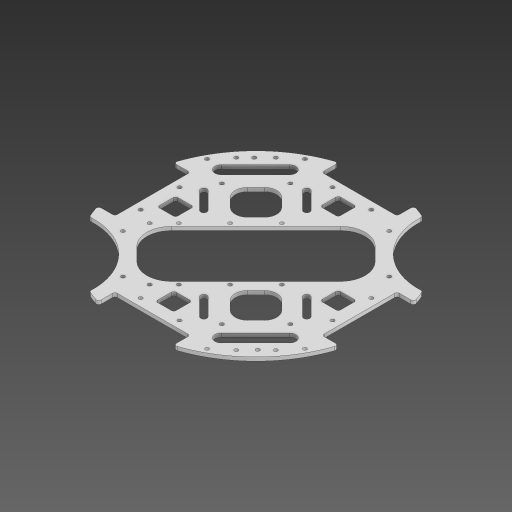
# Autodesk Inventor part: top
Saved by Autodesk Inventor 2023 (Build 270158000, 158)
## iProperties
Created: 2025-06-24
Part Number: top
Material: Типовые
Document SubType Name: Modeling
Designer: daa
Density: 1 g/cm^3
Appearance: По умолчанию
Author: daa
Autodesk Inventor part; units mm, degrees
ref_plane "YZ Plane" through (0, 0, 0) normal (1, 0, 0) x (0, 1, 0)
ref_plane "XZ Plane" through (0, 0, 0) normal (0, 1, 0) x (-1, 0, 0)
ref_plane "XY Plane" through (0, 0, 0) normal (0, 0, 1) x (1, 0, 0)
sketch "Эскиз1" plane through (0, 0, 0) normal (0, 1, 0) x (-1, 0, 0)
  line L0 (-79, -47.2724) -> (-79, 14.7276)
  line L1 (91.5447, -47.2724) -> (91.5447, 14.7276)
  line L2 (-79, -47.2724) -> (-93, -47.2724)
  line L3 (-79, 14.7276) -> (-93, 14.7276)
  line L4 (91.5447, -47.2724) -> (105.5447, -47.2724)
  line L5 (91.5447, 14.7276) -> (105.5447, 14.7276)
  line L6 (-24.7276, -101.5447) -> (37.2724, -101.5447)
  line L7 (-24.7276, 69) -> (37.2724, 69)
  line L8 (-24.7276, 69) -> (-24.7276, 83)
  line L9 (37.2724, 69) -> (37.2724, 83)
  line L10 (37.2724, -101.5447) -> (37.2724, -115.5447)
  line L11 (-24.7276, -101.5447) -> (-24.7276, -115.5447)
  arc A0 (-93, -47.2724) -> (-24.7276, -115.5447) centre (6.2724, -16.2724) ccw
  arc A1 (105.5447, 14.7276) -> (37.2724, 83) centre (6.2724, -16.2724) ccw
  arc A2 (-24.7276, 83) -> (-93, 14.7276) centre (6.2724, -16.2724) ccw
  arc A3 (37.2724, -115.5447) -> (105.5447, -47.2724) centre (6.2724, -16.2724) ccw
  dimension "d29" = 62
  dimension "d31" = 62
  dimension "d33" = 14
  dimension "d34" = 14
  dimension "d35" = 62
  dimension "d36" = 62
  dimension "d39" = 14
  dimension "d40" = 14
  constraints: 24 end point, 8 point on circle, 4 centre point, 4 horizontal, 3 parallel, 3 vertical, 2 point on line, 1 concentric
  measures "d29" distance of L0.start L0.end
  measures "d31" distance of L1.start L1.end
  measures "d33" distance of L0.end L3.end
  measures "d34" distance of L1.end L5.end
  measures "d35" distance of L6.start L6.end
  measures "d36" distance of L7.start L7.end
  measures "d39" distance of L7.start L8.end
  measures "d40" distance of L6.start L11.end
extrude "motor" add sketch "Эскиз1" along normal blind 3
sketch "Эскиз2" plane through (0, 3, 0) normal (0, 1, 0) x (1, 0, 0)
  arc A0 (24.7276, -83) -> (93, -14.7276) centre (-6.2724, 16.2724) ccw projected
  arc A1 (-37.2724, 115.5447) -> (-105.5447, 47.2724) centre (-6.2724, 16.2724) ccw projected
  circle A2 centre (-6.2724, 16.2724) radius 104
  line L0 (-6.2724, 16.2724) -> (-6.2724, -50.7276)
  arc A3 (-37.2724, 115.5447) -> (-105.5447, 47.2724) centre (-6.2724, 16.2724) ccw projected
  line L1 (-88.7917, -14.3063) -> (-40.8426, -62.2554)
  line L2 (-101.3809, -25.8032) -> (-48.3479, -78.8362)
  arc A4 (-105.5447, -14.7276) -> (-37.2724, -83) centre (-6.2724, 16.2724) ccw projected
  arc A5 (-48.3479, -78.8362) -> (-101.3809, -25.8032) centre (-98.035, -75.4903) ccw
  arc A6 (24.7276, -83) -> (93, -14.7276) centre (-6.2724, 16.2724) ccw projected
  line L3 (-79.8115, 89.8115) -> (67.2668, -57.2668)
  line L4 (24.3063, 98.7917) -> (72.2554, 50.8426)
  line L5 (35.8032, 111.3809) -> (88.8362, 58.3479)
  arc A7 (93, 47.2724) -> (24.7276, 115.5447) centre (-6.2724, 16.2724) ccw
  arc A8 (35.8032, 111.3809) -> (88.8362, 58.3479) centre (85.4903, 108.035) ccw
  line L6 (-91.5447, -14.7276) -> (-105.5447, -14.7276) projected
  arc A9 (-105.5447, -14.7276) -> (-101.3809, -25.8032) centre (-6.2724, 16.2724) ccw
  line L7 (-105.5447, -14.7276) -> (-80, -14.7276)
  point P0 (0, 0)
  point P1 (-6.2724, -50.7276)
  dimension "d181" = 208
  dimension "d190" = 67
  dimension "d205" = 75
  dimension "d207" = 17.0315
  dimension "d208" = 11.0756
  dimension "d209" = 104
  constraints: 14 end point, 10 point on circle, 7 symmetric about line, 5 centre point, 2 tangent, 1 point on line, 1 vertical, 2 other
  measures "d181" diameter of A2
  measures "d190" distance of L0.end L0.start
  measures "d205" distance of L2.start L2.end
  measures "d207" distance between parallel lines of L1 L2
  measures "d208" horizontal distance of A2.end L2.end
  measures "d209" radius of A9
extrude "ball" cut sketch "Эскиз2" against normal blind 3 contours A2 L2 | L2 A5 | L5 A2 | A8 L5
sketch "Эскиз3" plane through (0, 3, 0) normal (0, 1, 0) x (1, 0, 0)
  arc A0 (93, 47.2724) -> (24.7276, 115.5447) centre (-6.2724, 16.2724) ccw projected
  line L0 (-6.2724, 16.2724) -> (97.7276, 16.2724) construction
  line L1 (67.2668, 89.8115) -> (-62.5447, -40)
  circle A1 centre (70.5306, -44.2673) radius 1.5
  circle A2 centre (54.2672, -60.5308) radius 1.5
  circle A3 centre (41.3053, -71.6104) radius 1.5
  circle A4 centre (81.6104, -31.3053) radius 1.5
  arc A5 (24.7276, -83) -> (93, -14.7276) centre (-6.2724, 16.2724) ccw projected
  line L2 (-6.2724, 16.2724) -> (97.7276, 16.2724) construction
  line L3 (-79.8115, 89.8115) -> (67.2668, -57.2668)
  line L4 (-91.5447, 47.2724) -> (-91.5447, -14.7276) projected
  line L5 (-91.5447, 16.2724) -> (79, 16.2724)
  line L6 (24.7276, 101.5447) -> (-37.2724, 101.5447) projected
  line L7 (-6.2724, 101.5447) -> (-6.2724, -69)
  line L8 (-6.2724, 101.5447) -> (-6.2724, -69)
  line L9 (-91.5447, 47.2724) -> (-91.5447, -14.7276) projected
  arc A6 (24.7276, -83) -> (93, -14.7276) centre (-6.2724, 16.2724) ccw projected
  circle A7 centre (-66.812, 93.0753) radius 1.5
  circle A8 centre (-83.0755, 76.8119) radius 1.5
  circle A9 centre (-94.1551, 63.85) radius 1.5
  circle A10 centre (-53.85, 104.1551) radius 1.5
  point P0 (0, 0)
  point P1 (67.2668, -57.2668)
  point P2 (67.2668, -57.2668)
  point P3 (-105.5447, 47.2724)
  point P4 (-79.8115, 89.8115)
  point P5 (-79.8115, 89.8115)
  point P6 (-79.8115, 89.8115)
  dimension "d65" = 3
  dimension "d66" = 3
  dimension "d67" = 3
  dimension "d68" = 3
  dimension "d69" = 23
  dimension "d71" = 57
  dimension "d74" = -12.962
  dimension "d78" = 25.9614
  constraints: 14 end point, 8 centre point, 8 symmetric about line, 4 point on circle, 3 midpoint, 2 horizontal, 2 vertical, 1 point on line, 4 other
  measures "d65" diameter of A1
  measures "d66" diameter of A2
  measures "d67" diameter of A3
  measures "d68" diameter of A4
  measures "d69" distance of A2.centre A1.centre
  measures "d71" distance of A3.centre A4.centre
  measures "d74" vertical distance of A1.centre A4.centre
  measures "d78" vertical distance of A4.centre point (67.267, -57.267)
extrude "hand_mount" cut sketch "Эскиз3" against normal blind 10
sketch "Эскиз5" plane through (0, 3, 0) normal (0, 1, 0) x (1, 0, 0)
  circle A0 centre (29.7645, -47.992) radius 1.5
  circle A1 centre (58.0485, -19.7074) radius 1.5
  circle A2 centre (-6.2982, 16.355) radius 104
  arc A3 (-105.5447, -14.7276) -> (-99.04, -30.7083) centre (-6.2982, 16.355) ccw projected
  line L0 (-6.2982, 16.355) -> (97.7018, 16.355) construction
  line L1 (67.2409, 89.8941) -> (-79.8373, -57.1841)
  circle A4 centre (-70.6452, 52.4178) radius 1.5
  circle A5 centre (-42.3607, 80.7017) radius 1.5
  circle A6 centre (-44.9008, -54.7745) radius 1.5
  line L2 (-46.7704, -39.7817) -> (-62, -24)
  arc A7 (-53.253, -76.4953) -> (-99.04, -30.7083) centre (-88.8109, -66.2662) ccw projected
  line L3 (-62.7022, -40.049) -> (-61.1643, -38.511)
  line L4 (-61.1643, -38.511) -> (-44.8852, -38.511) construction
  line L5 (-61.1643, -38.511) -> (-44.9008, -54.7745)
  circle A8 centre (-77.4277, -22.2476) radius 1.5
  arc A9 (24.7276, -83) -> (93, -14.7276) centre (-6.2724, 16.2724) ccw projected
  line L6 (-6.2982, 16.355) -> (97.7785, 16.355) construction
  line L7 (67.2952, -57.2383) -> (-79.783, 89.8399)
  arc A10 (-37.2724, 115.5447) -> (-105.5447, 47.2724) centre (-6.2724, 16.2724) ccw projected
  circle A11 centre (64.8313, 54.9576) radius 1.5
  circle A12 centre (32.3044, 87.4845) radius 1.5
  point P0 (0, 0)
  dimension "d119" = 208
  dimension "d116" = 3
  dimension "d117" = 3
  dimension "d118" = 40
  dimension "d121" = 64.347
  dimension "d126" = 3
  dimension "d130" = 2.175
  dimension "d133" = 23
  constraints: 16 end point, 8 centre point, 5 symmetric about line, 4 point on circle, 3 horizontal, 2 point on line, 1 coincident, 9 other
  measures "d116" diameter of A0
  measures "d117" diameter of A1
  measures "d118" distance of A1.centre A0.centre
  measures "d121" vertical distance of L0.start A0.centre
  measures "d126" diameter of A6
  measures "d130" distance of L3.start L3.end
  measures "d133" distance of L3.end L5.end
extrude "Выдавливание5" cut sketch "Эскиз5" against normal blind 10 contours A0 | A1 | A4 | A5 | A6 | A8 | A11 | A12
sketch "Эскиз6" plane through (0, 3, 0) normal (0, 1, 0) x (1, 0, 0)
  circle A0 centre (-22.2724, 95.2947) radius 1.5
  circle A1 centre (9.7276, 95.2947) radius 1.5
  line L0 (24.7276, 115.5447) -> (24.7276, 101.5447) projected
  line L1 (24.7276, 101.5447) -> (-37.2724, 101.5447) projected
  circle A2 centre (-22.2724, -62.75) radius 1.5
  circle A3 centre (9.7276, -62.75) radius 1.5
  circle A4 centre (-85.2947, 32.2724) radius 1.5
  circle A5 centre (-85.2947, 0.2724) radius 1.5
  circle A6 centre (72.75, 32.2724) radius 1.5
  circle A7 centre (72.75, 0.2724) radius 1.5
  point P0 (0, 0)
  point P1 (24.7276, -69)
  point P2 (-37.2724, -69)
  point P3 (-91.5447, -14.7276)
  point P4 (-91.5447, 47.2724)
  point P5 (79, 47.2724)
  point P6 (79, -14.7276)
  dimension "d135" = 3
  dimension "d136" = 3
  dimension "d137" = 32
  dimension "d138" = 15
  dimension "d139" = 6.25
  dimension "d140" = 3
  dimension "d141" = 3
  dimension "d142" = 6.25
  dimension "d143" = 32
  dimension "d144" = 15
  dimension "d145" = 6.25
  dimension "d146" = 6.25
  dimension "d147" = 3
  dimension "d148" = 3
  dimension "d149" = 32
  dimension "d150" = 15
  dimension "d151" = 6.25
  dimension "d152" = 6.25
  dimension "d153" = 3
  dimension "d154" = 3
  dimension "d155" = 32
  dimension "d156" = 15
  dimension "d157" = 6.25
  dimension "d158" = 6.25
  constraints: 8 centre point
  measures "d135" diameter of A0
  measures "d136" diameter of A1
  measures "d137" distance of A1.centre A0.centre
  measures "d138" distance from line of L0 A1.centre
  measures "d139" distance from line of L1 A1.centre
  measures "d140" diameter of A2
  measures "d141" diameter of A3
  measures "d142" distance from line of L1 A0.centre
  measures "d143" distance of A2.centre A3.centre
  measures "d144" horizontal distance of point (24.728, -69) A3.centre
  measures "d145" vertical distance of point (24.728, -69) A3.centre
  measures "d146" vertical distance of point (-37.272, -69) A2.centre
  measures "d147" diameter of A4
  measures "d148" diameter of A5
  measures "d149" distance of A5.centre A4.centre
  measures "d150" vertical distance of A5.centre point (-91.545, -14.728)
  measures "d151" horizontal distance of A5.centre point (-91.545, -14.728)
  measures "d152" horizontal distance of A4.centre point (-91.545, 47.272)
  measures "d153" diameter of A6
  measures "d154" diameter of A7
  measures "d155" distance of A7.centre A6.centre
  measures "d156" vertical distance of point (79, 47.272) A6.centre
  measures "d157" horizontal distance of point (79, -14.728) A7.centre
  measures "d158" horizontal distance of point (79, 47.272) A6.centre
extrude "Выдавливание6" cut sketch "Эскиз6" against normal blind 10
fillet "Сопряжение1" radius 2 20 edges at (88.8362, 1.5, -58.3479) (35.8032, 1.5, -111.3809) (93, 1.5, -47.2724) (24.7276, 1.5, -115.5447) (24.7276, 1.5, -101.5447) (-37.2724, 1.5, -101.5447) (-37.2724, 1.5, -115.5447) (-105.5447, 1.5, -47.2724) (-91.5447, 1.5, -47.2724) (-91.5447, 1.5, 14.7276) (-105.5447, 1.5, 14.7276) (-48.3479, 1.5, 78.8362) (-101.3809, 1.5, 25.8032) (-37.2724, 1.5, 83) (-37.2724, 1.5, 69) (24.7276, 1.5, 69) (24.7276, 1.5, 83) (93, 1.5, 14.7276) (79, 1.5, 14.7276) (79, 1.5, -47.2724)
fillet_without_effect "Сопряжение4"
sketch "Эскиз8" plane through (0, 3, 0) normal (0, 1, 0) x (1, 0, 0)
  circle A0 centre (-75.6509, 84.2365) radius 1.6
  circle A1 centre (62.8514, -51.4283) radius 1.6
  circle A2 centre (-83.0755, 76.8119) radius 1.5
  circle A3 centre (-83.0755, 76.8119) radius 1.5 projected
  line L0 (-83.0755, 76.8119) -> (-75.6509, 84.2365)
  line L1 (-83.0755, 76.8119) -> (-72.5755, 76.8119) construction
  circle A4 centre (54.2672, -60.5308) radius 1.5
  circle A5 centre (54.2672, -60.5308) radius 1.5 projected
  line L2 (54.2672, -60.5308) -> (67.7672, -60.5308) construction
  circle A6 centre (70.5306, -44.2673) radius 1.5
  circle A7 centre (70.5306, -44.2673) radius 1.5 projected
  line L3 (70.5306, -44.2673) -> (62.8514, -51.4283)
  line L4 (70.5306, -44.2673) -> (81.0306, -44.2673) construction
  point P0 (0, 0)
  dimension "d211" = 3.2
  dimension "d212" = 3.2
  dimension "d213" = 3
  dimension "d214" = 10.5
  dimension "d215" = 45
  dimension "d216" = 3
  dimension "d221" = 3
  dimension "d222" = 10.5
  dimension "d223" = 137
  constraints: 10 end point, 5 centre point, 3 concentric, 3 horizontal, 2 coincident, 2 equal length
  measures "d211" diameter of A0
  measures "d212" diameter of A1
  measures "d213" diameter of A2
  measures "d214" distance of L0.start L0.end
  measures "d215" angle of L1 L0
  measures "d216" diameter of A4
  measures "d221" diameter of A6
  measures "d222" distance of L3.start L3.end
  measures "d223" angle of L3 L4
extrude "Выдавливание7" cut sketch "Эскиз8" against normal blind 10 contours A0 | A1
sketch "Эскиз9" plane through (0, 3, 0) normal (0, 1, 0) x (1, 0, 0)
  line L0 (-38.87, 27.5154) -> (-17.5154, 48.87)
  line L1 (-17.5154, 48.87) -> (26.3253, 5.0294)
  line L2 (26.3253, 5.0294) -> (4.9706, -16.3253)
  line L3 (4.9706, -16.3253) -> (-38.87, 27.5154)
  circle A0 centre (-6.2724, 16.2724) radius 104
  arc A1 (-39.9194, 114.679) -> (-104.679, 49.9194) centre (-6.2724, 16.2724) ccw projected
  circle A2 centre (-17.5154, 48.87) radius 1.5
  circle A3 centre (-38.87, 27.5154) radius 1.5
  circle A4 centre (4.9706, -16.3253) radius 1.5
  circle A5 centre (26.3253, 5.0294) radius 1.5
  point P0 (0, 0)
  dimension "d224" = 30.2
  dimension "d225" = 62
  dimension "d226" = 208
  dimension "d227" = 15.1
  dimension "d229" = 31
  dimension "d230" = 3
  dimension "d231" = 3
  dimension "d232" = 3
  dimension "d233" = 3
  constraints: 8 end point, 5 centre point, 4 coincident, 2 parallel, 1 concentric, 1 perpendicular
  measures "d224" distance of L1.end L2.end
  measures "d225" distance of L0.end L1.end
  measures "d226" diameter of A0
  measures "d227" distance from line of L1 A0.centre
  measures "d229" distance from line of L2 A0.centre
  measures "d230" diameter of A2
  measures "d231" diameter of A3
  measures "d232" diameter of A4
  measures "d233" diameter of A5
extrude "Выдавливание8" cut sketch "Эскиз9" against normal blind 10 contours L3 A3 L0 | L0 A3 L3 | A2 L1 L0 | L0 L1 A2 | A4 L2 L3 | L3 L2 A4 | A5 L2 L1 | L1 L2 A5
sketch "Эскиз10" plane through (0, 3, 0) normal (0, 1, 0) x (1, 0, 0)
  circle A0 centre (-6.2724, 16.2719) radius 104.0005
  arc A1 (-39.9194, 114.679) -> (-104.679, 49.9194) centre (-6.2724, 16.2724) ccw projected
  line L0 (-60.0125, 6.3729) -> (-72.0333, -5.648)
  line L1 (-72.0333, -5.648) -> (-28.1927, -49.4886)
  line L2 (-28.1927, -49.4886) -> (-16.1718, -37.4678)
  line L3 (-16.1718, -37.4678) -> (-60.0125, 6.3729)
  circle A2 centre (-60.0125, 6.3729) radius 1.5
  circle A3 centre (-72.0333, -5.648) radius 1.5
  circle A4 centre (-16.1718, -37.4678) radius 1.5
  circle A5 centre (-28.1927, -49.4886) radius 1.5
  point P0 (0, 0)
  dimension "d248" = 17
  dimension "d249" = 62
  dimension "d250" = 9.899
  dimension "d251" = 45
  dimension "d252" = 3
  dimension "d253" = 3
  dimension "d254" = 3
  dimension "d255" = 3
  constraints: 8 end point, 5 centre point, 4 coincident, 2 parallel, 1 perpendicular, 1 tangent
  measures "d248" distance of L2.end L1.end
  measures "d249" distance of L1.end L0.end
  measures "d250" vertical distance of L0.start A0.centre
  measures "d251" distance from line of L3 A1.centre
  measures "d252" diameter of A2
  measures "d253" diameter of A3
  measures "d254" diameter of A4
  measures "d255" diameter of A5
extrude "Выдавливание9" cut sketch "Эскиз10" against normal blind 10 contours L3 A2 L0 | L0 A2 L3 | A3 L1 L0 | L0 L1 A3 | A4 L2 L3 | L3 L2 A4 | A5 L2 L1 | L1 L2 A5
sketch "Эскиз12" plane through (0, 3, 0) normal (0, 1, 0) x (1, 0, 0)
  line L0 (-49.8565, -38.2721) -> (-60.8166, -27.3119)
  line L1 (-60.8166, 0.9723) -> (9.0278, 70.8168)
  line L2 (37.3121, 70.8168) -> (48.2723, 59.8566)
  line L3 (48.2723, 31.5724) -> (-21.5722, -38.2721)
  circle A0 centre (-6.2724, 16.2724) radius 104
  arc A1 (27.3747, -82.1343) -> (92.1343, -17.3747) centre (-6.2724, 16.2724) ccw projected
  arc A2 (48.2723, 31.5724) -> (48.2723, 59.8566) centre (34.1301, 45.7145) ccw
  arc A3 (37.3121, 70.8168) -> (9.0278, 70.8168) centre (23.17, 56.6747) ccw
  arc A4 (-60.8166, 0.9723) -> (-60.8166, -27.3119) centre (-46.6745, -13.1698) ccw
  arc A5 (-49.8565, -38.2721) -> (-21.5722, -38.2721) centre (-35.7144, -24.13) ccw
  line L4 (-91.5447, 45.2724) -> (-91.5447, -12.7276) projected
  line L5 (-91.5447, 45.2724) -> (-91.5447, -12.7276) projected
  line L6 (79, -12.7276) -> (79, 45.2724) projected
  line L7 (22.7276, 101.5447) -> (-35.2724, 101.5447) projected
  line L8 (-35.2724, -69) -> (22.7276, -69) projected
  line L9 (-57.1845, 60.113) -> (-50.1134, 67.184)
  line L10 (-35.9713, 67.184) -> (-28.9002, 60.113)
  line L11 (-28.9002, 45.9708) -> (-35.9713, 38.8998)
  line L12 (-50.1134, 38.8998) -> (-57.1845, 45.9708)
  arc A6 (-57.1845, 60.113) -> (-57.1845, 45.9708) centre (-50.1134, 53.0419) ccw
  arc A7 (-35.9713, 67.184) -> (-50.1134, 67.184) centre (-43.0424, 60.113) ccw
  arc A8 (-28.9002, 45.9708) -> (-28.9002, 60.113) centre (-35.9713, 53.0419) ccw
  arc A9 (-50.1134, 38.8998) -> (-35.9713, 38.8998) centre (-43.0424, 45.9708) ccw
  line L13 (79, 16.2724) -> (-91.5447, 16.2724)
  line L14 (-6.2724, 101.5447) -> (-6.2724, -69)
  arc A10 (-48.275, -77.4757) -> (-100.0204, -25.7303) centre (-98.035, -75.4903) ccw projected
  line L15 (-6.2724, 16.2724) -> (73.7, 16.2724) construction
  line L16 (-62.8214, -40.2767) -> (50.2767, 72.8214)
  arc A11 (35.7303, 110.0204) -> (87.4757, 58.275) centre (85.4903, 108.035) ccw projected
  line L17 (37.5683, -34.6398) -> (44.6393, -27.5687)
  line L18 (44.6393, -13.4266) -> (37.5683, -6.3555)
  line L19 (23.4261, -6.3555) -> (16.3551, -13.4266)
  line L20 (16.3551, -27.5687) -> (23.4261, -34.6398)
  arc A12 (23.4261, -34.6398) -> (37.5683, -34.6398) centre (30.4972, -27.5687) ccw
  arc A13 (44.6393, -27.5687) -> (44.6393, -13.4266) centre (37.5683, -20.4976) ccw
  arc A14 (37.5683, -6.3555) -> (23.4261, -6.3555) centre (30.4972, -13.4266) ccw
  arc A15 (16.3551, -13.4266) -> (16.3551, -27.5687) centre (23.4261, -20.4976) ccw
  line L21 (-80.6868, 61.9019) -> (-52.4026, 90.1862) construction
  line L22 (-77.1513, 58.3663) -> (-48.867, 86.6506)
  line L23 (-55.9381, 93.7217) -> (-84.2224, 65.4374)
  arc A16 (-84.2224, 65.4374) -> (-77.1513, 58.3663) centre (-80.6868, 61.9019) ccw
  arc A17 (-48.867, 86.6506) -> (-55.9381, 93.7217) centre (-52.4026, 90.1862) ccw
  line L24 (-80.6868, 61.9019) -> (-40.6868, 61.9019) construction
  line L25 (35.8216, -54.6066) -> (64.1059, -26.3223)
  line L26 (71.177, -33.3934) -> (42.8927, -61.6777)
  arc A18 (35.8216, -54.6066) -> (42.8927, -61.6777) centre (39.3572, -58.1421) ccw
  arc A19 (71.177, -33.3934) -> (64.1059, -26.3223) centre (67.6414, -29.8579) ccw
  point P0 (0, 0)
  point P1 (-35.7144, -52.4142)
  point P2 (23.17, 84.9589)
  point P3 (-74.9588, -13.1698)
  point P4 (62.4144, 45.7145)
  point P5 (-21.8291, 53.0419)
  point P6 (-43.0424, 74.2551)
  point P7 (-43.0424, 31.8287)
  point P8 (51.7104, -20.4976)
  point P9 (-66.5447, 76.044)
  dimension "d256" = 55.5
  dimension "d257" = 138.775
  dimension "d258" = 208
  dimension "d260" = -29.4422
  dimension "d261" = 20
  dimension "d271" = 30
  dimension "d272" = 30
  dimension "d274" = 36.7696
  dimension "d275" = 10
  dimension "d276" = 10
  dimension "d278" = 40
  dimension "d279" = 45
  dimension "d280" = 10
  dimension "d281" = 25
  constraints: 46 end point, 34 point on circle, 21 tangent, 19 symmetric about line, 17 centre point, 16 point on line, 5 equal radius, 5 midpoint, 5 parallel, 2 horizontal, 2 perpendicular, 1 equal length, 6 other
  measures "d256" distance of point (23.17, 84.959) point (62.414, 45.715)
  measures "d257" distance of point (-74.959, -13.17) point (23.17, 84.959)
  measures "d258" diameter of A0
  measures "d260" vertical distance of point (-74.959, -13.17) L15.start
  measures "d261" radius of A2
  measures "d271" distance of point (-21.829, 53.042) point (-43.042, 31.829)
  measures "d272" distance of point (-43.042, 74.255) point (-21.829, 53.042)
  measures "d274" vertical distance of A0.centre point (-21.829, 53.042)
  measures "d275" radius of A6
  measures "d276" radius of A9
  measures "d278" distance of L21.start L21.end
  measures "d279" angle of L24 L21
  measures "d280" diameter of A17
  measures "d281" distance from line of L4 point (-66.545, 76.044)
extrude "Выдавливание10" cut sketch "Эскиз12" against normal blind 10 contours L0 L16 L14 L3 A5 | L0 A4 L1 L13 L16 | L16 L2 A2 L3 L13 | L13 L1 L14 | L13 L3 L14 | L14 L1 A3 L2 L16 | L9 A7 L10 A8 L11 A9 L12 A6 | A12 L20 A15 L19 A14 L18 A13 L17 | A16 L23 A17 L22 | L25 A19 L26 A18
sketch "Эскиз13" plane through (0, 3, 0) normal (0, 1, 0) x (1, 0, 0)
  circle A0 centre (-6, 17) radius 104
  line L0 (-11.7724, 91.5447) -> (-0.7724, 91.5447)
  line L1 (1.2276, 89.5447) -> (1.2276, 78.5447)
  line L2 (-0.7724, 76.5447) -> (-11.7724, 76.5447)
  line L3 (-13.7724, 78.5447) -> (-13.7724, 89.5447)
  line L4 (22.7276, 101.5447) -> (-35.2724, 101.5447) projected
  line L5 (-110, 17) -> (98, 17)
  line L6 (-0.7724, -44) -> (-11.7724, -44)
  line L7 (-13.7724, -46) -> (-13.7724, -57)
  line L8 (-11.7724, -59) -> (-0.7724, -59)
  line L9 (1.2276, -57) -> (1.2276, -46)
  line L10 (-35.2724, -69) -> (22.7276, -69) projected
  line L11 (-6, 17) -> (-79.5391, -56.5391)
  line L12 (-6, 17) -> (98, 17) construction
  line L13 (-79.5391, -56.5391) -> (67.5391, 90.5391)
  line L14 (68.5447, 11.2276) -> (68.5447, 22.2276)
  line L15 (66.5447, 24.2276) -> (55.5447, 24.2276)
  line L16 (53.5447, 22.2276) -> (53.5447, 11.2276)
  line L17 (55.5447, 9.2276) -> (66.5447, 9.2276)
  line L18 (-6, 17) -> (-6, 121)
  line L19 (-6, -87) -> (-6, 121)
  line L20 (-67.5447, 9.2276) -> (-78.5447, 9.2276)
  line L21 (-80.5447, 11.2276) -> (-80.5447, 22.2276)
  line L22 (-78.5447, 24.2276) -> (-67.5447, 24.2276)
  line L23 (-65.5447, 22.2276) -> (-65.5447, 11.2276)
  arc A1 (-78.5447, 24.2276) -> (-80.5447, 22.2276) centre (-78.5447, 22.2276) ccw
  arc A2 (-65.5447, 22.2276) -> (-67.5447, 24.2276) centre (-67.5447, 22.2276) ccw
  arc A3 (-67.5447, 9.2276) -> (-65.5447, 11.2276) centre (-67.5447, 11.2276) ccw
  arc A4 (-80.5447, 11.2276) -> (-78.5447, 9.2276) centre (-78.5447, 11.2276) ccw
  arc A5 (-11.7724, 91.5447) -> (-13.7724, 89.5447) centre (-11.7724, 89.5447) ccw
  arc A6 (-13.7724, 78.5447) -> (-11.7724, 76.5447) centre (-11.7724, 78.5447) ccw
  arc A7 (-0.7724, 76.5447) -> (1.2276, 78.5447) centre (-0.7724, 78.5447) ccw
  arc A8 (1.2276, 89.5447) -> (-0.7724, 91.5447) centre (-0.7724, 89.5447) ccw
  arc A9 (-11.7724, -44) -> (-13.7724, -46) centre (-11.7724, -46) ccw
  arc A10 (1.2276, -46) -> (-0.7724, -44) centre (-0.7724, -46) ccw
  arc A11 (-13.7724, -57) -> (-11.7724, -59) centre (-11.7724, -57) ccw
  arc A12 (-0.7724, -59) -> (1.2276, -57) centre (-0.7724, -57) ccw
  arc A13 (53.5447, 11.2276) -> (55.5447, 9.2276) centre (55.5447, 11.2276) ccw
  arc A14 (55.5447, 24.2276) -> (53.5447, 22.2276) centre (55.5447, 22.2276) ccw
  arc A15 (68.5447, 22.2276) -> (66.5447, 24.2276) centre (66.5447, 22.2276) ccw
  arc A16 (66.5447, 9.2276) -> (68.5447, 11.2276) centre (66.5447, 11.2276) ccw
  line L24 (-73.0447, 40) -> (-58.9026, 25.8579) construction
  line L25 (-74.8125, 38.2322) -> (-60.6703, 24.0901)
  line L26 (-57.1348, 27.6256) -> (-71.2769, 41.7678)
  arc A17 (-71.2769, 41.7678) -> (-74.8125, 38.2322) centre (-73.0447, 40) ccw
  arc A18 (-60.6703, 24.0901) -> (-57.1348, 27.6256) centre (-58.9026, 25.8579) ccw
  line L27 (-73.0447, 40) -> (-53.0447, 40) construction
  line L28 (17, -50.0447) -> (2.8579, -35.9026) construction
  line L29 (15.2322, -51.8125) -> (1.0901, -37.6703)
  line L30 (4.6256, -34.1348) -> (18.7678, -48.2769)
  arc A19 (15.2322, -51.8125) -> (18.7678, -48.2769) centre (17, -50.0447) ccw
  arc A20 (4.6256, -34.1348) -> (1.0901, -37.6703) centre (2.8579, -35.9026) ccw
  line L31 (17, -50.0447) -> (17, -30.0447) construction
  line L32 (-73.0447, 40) -> (-30.6183, 82.4264)
  line L33 (-30.6183, 82.4264) -> (-16.4762, 68.2843) construction
  line L34 (-32.3861, 80.6586) -> (-18.2439, 66.5165)
  line L35 (-14.7084, 70.052) -> (-28.8505, 84.1942)
  arc A21 (-28.8505, 84.1942) -> (-32.3861, 80.6586) centre (-30.6183, 82.4264) ccw
  arc A22 (-18.2439, 66.5165) -> (-14.7084, 70.052) centre (-16.4762, 68.2843) ccw
  line L36 (-30.6183, 82.4264) -> (-10.6183, 82.4264) construction
  line L37 (57.6586, -9.3861) -> (43.5165, 4.7561)
  line L38 (47.052, 8.2916) -> (61.1942, -5.8505)
  arc A23 (57.6586, -9.3861) -> (61.1942, -5.8505) centre (59.4264, -7.6183) ccw
  arc A24 (47.052, 8.2916) -> (43.5165, 4.7561) centre (45.2843, 6.5238) ccw
  point P0 (0, 0)
  point P1 (-13.7724, 91.5447)
  point P2 (1.2276, 76.5447)
  point P3 (1.2276, 91.5447)
  point P4 (-13.7724, 76.5447)
  point P5 (-13.7724, -59)
  point P6 (-13.7724, -44)
  point P7 (1.2276, -59)
  point P8 (-6.2724, -69)
  point P9 (1.2276, -51.5)
  point P10 (68.5447, 9.2276)
  point P11 (53.5447, 24.2276)
  point P12 (68.5447, 24.2276)
  point P13 (53.5447, 9.2276)
  point P14 (-65.5447, 9.2276)
  point P15 (-65.5447, 24.2276)
  point P16 (-80.5447, 9.2276)
  point P17 (-80.5447, 24.2276)
  point P18 (-65.9736, 32.9289)
  point P19 (9.9289, -42.9736)
  point P20 (-23.5472, 75.3553)
  dimension "d282" = 208
  dimension "d283" = 15
  dimension "d284" = 15
  dimension "d285" = 10
  dimension "d286" = 21.5
  dimension "d287" = 15
  dimension "d288" = 15
  dimension "d289" = 10
  dimension "d290" = 21.5
  dimension "d291" = 135
  dimension "d292" = 2
  dimension "d295" = 20
  dimension "d296" = 45
  dimension "d297" = 5
  dimension "d298" = 60
  dimension "d299" = 20
  dimension "d300" = 45
  dimension "d301" = 5
  constraints: 80 end point, 48 point on circle, 40 tangent, 32 point on line, 24 centre point, 22 symmetric about line, 15 equal radius, 6 parallel, 5 horizontal, 4 midpoint, 3 equal length, 2 perpendicular, 1 vertical, 13 other
  measures "d283" distance of point (1.228, 76.545) point (-13.772, 76.545)
  measures "d284" distance of point (1.228, 91.545) point (1.228, 76.545)
  measures "d285" distance between parallel lines of L4 L0
  measures "d286" distance from line of L4.start L1
  measures "d287" distance of point (1.228, -59) point (-13.772, -59)
  measures "d288" distance of point (-13.772, -59) point (-13.772, -44)
  measures "d289" distance from line of point (-6.272, -69) L8
  measures "d290" horizontal distance of L10.end point (1.228, -51.5)
  measures "d291" angle of L11 L12
  measures "d292" radius of A1
  measures "d295" distance of L24.start L24.end
  measures "d296" angle of L24 L27
  measures "d297" diameter of A18
  measures "d298" distance of L24.start L32.end
  measures "d299" distance of L32.end L33.end
  measures "d300" angle of L33 L36
  measures "d301" diameter of A22
extrude "Выдавливание11" cut sketch "Эскиз13" against normal blind 10 contours L14 A16 L17 A13 L16 L5 | L5 L16 A14 L15 A15 L14 | L23 A3 L20 A4 L21 L5 | L5 L21 A1 L22 A2 L23 | L18 L0 A8 L1 A7 L2 | L2 A6 L3 A5 L0 L18 | L19 L8 A11 L7 A9 L6 | L6 A10 L9 A12 L8 L19 | A17 L26 A18 L25 | L29 A20 L30 A19 | A21 L35 A22 L34 | L37 A24 L38 A23
